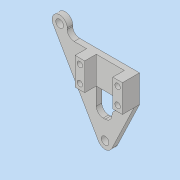
# Autodesk Inventor part: ribbonCableMount1
Saved by Autodesk Inventor 2017 (Build 210142000, 142)
## iProperties
Created: 2019-07-12
Part Number: ribbonCableMount1
Material: Generic
Document SubType Name: Modeling
Designer: techn
Density: 1 g/cm^3
Appearance: Default
Author: techn
Autodesk Inventor part; units mm, degrees
ref_plane "YZ Plane" through (0, 0, 0) normal (1, 0, 0) x (0, 1, 0)
ref_plane "XZ Plane" through (0, 0, 0) normal (0, 1, 0) x (-1, 0, 0)
ref_plane "XY Plane" through (0, 0, 0) normal (0, 0, 1) x (1, 0, 0)
sketch "Sketch1" plane through (0, 0, 0) normal (0, 0, 1) x (1, 0, 0)
  circle A0 centre (0, 0) radius 3.4925
  circle A1 centre (-20.955, 36.2951) radius 3.4925
  line L0 (0, 0) -> (-43.0857, 0) construction
  circle A2 centre (-20.955, 36.2951) radius 1.778
  circle A3 centre (0, 0) radius 1.778
  line L1 (-17.4625, 36.2951) -> (-17.4625, 32.4851)
  line L2 (-17.4625, 32.4851) -> (13.335, 32.4851)
  line L3 (13.335, 32.4851) -> (13.335, 19.7886)
  line L4 (13.335, 19.7886) -> (3.1507, -1.5068)
  line L5 (-23.9796, 34.5489) -> (-3.0246, -1.7463)
  dimension "d0" = 6.985
  dimension "d1" = 6.985
  dimension "d2" = 41.91
  dimension "d3" = 60
  dimension "d5" = 3.556
  dimension "d6" = 3.556
  dimension "d7" = 3.81
  dimension "d8" = 34.29
  constraints: 12 end point, 4 centre point, 4 point on circle, 4 tangent, 3 coincident, 2 perpendicular, 1 horizontal, 1 vertical
  measures "d0" diameter of A0
  measures "d1" diameter of A1
  measures "d2" distance of point (0, 0) A1.centre
  measures "d5" diameter of A2
  measures "d6" diameter of A3
  measures "d7" distance from line of L2 A1.centre
  measures "d8" distance from line of L3 A1.centre
extrude "Extrusion1" add sketch "Sketch1" along normal blind 2.54
sketch "Sketch3" plane through (0, 0, 2.54) normal (0, 0, 1) x (1, 0, 0)
  circle A0 centre (-20.955, 36.2951) radius 1.778 construction
  circle A1 centre (0, 0) radius 1.778 construction
  arc A2 (-3.0246, -1.7463) -> (3.1507, -1.5068) centre (0, 0) ccw construction
  line L0 (3.1507, -1.5068) -> (13.335, 19.7886) construction
  line L1 (13.335, 19.7886) -> (13.335, 32.4851) construction
  line L2 (13.335, 32.4851) -> (-17.4625, 32.4851) construction
  line L3 (-17.4625, 32.4851) -> (-17.4625, 36.2951) construction
  arc A3 (-17.4625, 36.2951) -> (-23.9796, 34.5489) centre (-20.955, 36.2951) ccw construction
  line L4 (-23.9796, 34.5489) -> (-3.0246, -1.7463) construction
  line L5 (13.335, 19.7886) -> (13.335, 32.4851) projected
  line L6 (13.335, 32.4851) -> (8.89, 32.4851)
  line L7 (8.89, 32.4851) -> (8.89, 19.7886)
  line L8 (8.89, 19.7886) -> (13.335, 19.7886)
  line L9 (13.335, 19.7886) -> (13.335, 32.4851)
  line L10 (-4.064, 32.4851) -> (-8.509, 32.4851)
  line L11 (-8.509, 32.4851) -> (-8.509, 19.7886)
  line L12 (-8.509, 19.7886) -> (-4.064, 19.7886)
  line L13 (-4.064, 19.7886) -> (-4.064, 32.4851)
  line L14 (8.89, 19.7886) -> (-4.064, 19.7886) construction
  dimension "d11" = 4.445
  dimension "d12" = 12.954
  constraints: 18 end point, 4 parallel, 2 collinear, 2 horizontal, 2 perpendicular, 2 point on line
  measures "d11" distance of L7.end L8.end
  measures "d12" distance between parallel lines of L13 L7
extrude "Extrusion2" add sketch "Sketch3" along normal blind 5.334
fillet "Fillet1" radius 3.175 1 edges at (-17.4625, 32.4851, 1.27)
sketch "Sketch4" plane through (0, 0, 2.54) normal (0, 0, 1) x (1, 0, 0)
  line L0 (-4.064, 32.4851) -> (-4.064, 19.7886) projected
  line L1 (-4.064, 19.7886) -> (8.89, 19.7886)
  line L2 (8.89, 19.7886) -> (8.89, 14.7086)
  line L3 (8.89, 14.7086) -> (-4.064, 14.7086)
  line L4 (-4.064, 14.7086) -> (-4.064, 19.7886)
  line L5 (-4.064, 14.7086) -> (3.175, 14.7086)
  line L6 (3.175, 14.7086) -> (3.175, 8.5581)
  line L7 (3.175, 8.5581) -> (-4.064, 8.5581)
  line L8 (-4.064, 8.5581) -> (-4.064, 14.7086)
  point P0 (0, 0)
  dimension "d16" = 5.08
  dimension "d17" = 7.239
  constraints: 16 end point, 4 parallel, 2 horizontal, 2 perpendicular
  measures "d16" distance of L1.end L2.end
  measures "d17" distance of L6.end L7.end
extrude "Extrusion3" cut sketch "Sketch4" against normal through all
fillet "Fillet2" radius 3.175 4 edges at (8.89, 14.7086, 1.27) (3.175, 8.5581, 1.27) (-4.064, 8.5581, 1.27) (3.175, 14.7086, 1.27)
sketch "Sketch5" plane through (0, 0, 7.874) normal (0, 0, 1) x (1, 0, 0)
  circle A0 centre (-6.2865, 29.9451) radius 1.27
  circle A1 centre (-6.2865, 22.3286) radius 1.27
  circle A2 centre (11.1125, 29.9451) radius 1.27
  circle A3 centre (11.1125, 22.3286) radius 1.27
  line L0 (-4.064, 32.4851) -> (-8.509, 32.4851) construction
  line L1 (-8.509, 32.4851) -> (-8.509, 19.7886) construction
  line L2 (-8.509, 19.7886) -> (-4.064, 19.7886) construction
  line L3 (-4.064, 19.7886) -> (-4.064, 32.4851) construction
  line L4 (13.335, 32.4851) -> (8.89, 32.4851) construction
  line L5 (8.89, 32.4851) -> (8.89, 19.7886) construction
  line L6 (8.89, 19.7886) -> (13.335, 19.7886) construction
  line L7 (13.335, 19.7886) -> (13.335, 32.4851) construction
  point P0 (0, 0)
  point P1 (-6.2865, 32.4851)
  point P2 (11.1125, 32.4851)
  dimension "d21" = 2.54
  dimension "d22" = 2.54
  dimension "d23" = 2.54
  dimension "d24" = 2.54
  dimension "d25" = 2.54
  dimension "d26" = 2.54
  constraints: 4 centre point, 4 vertical alignment, 2 horizontal alignment, 2 midpoint
  measures "d21" diameter of A0
  measures "d22" diameter of A1
  measures "d23" diameter of A2
  measures "d24" diameter of A3
  measures "d25" distance from line of L0 A0.centre
  measures "d26" distance from line of L2 A1.centre
extrude "Extrusion4" cut sketch "Sketch5" against normal through all
body "Solid1"
